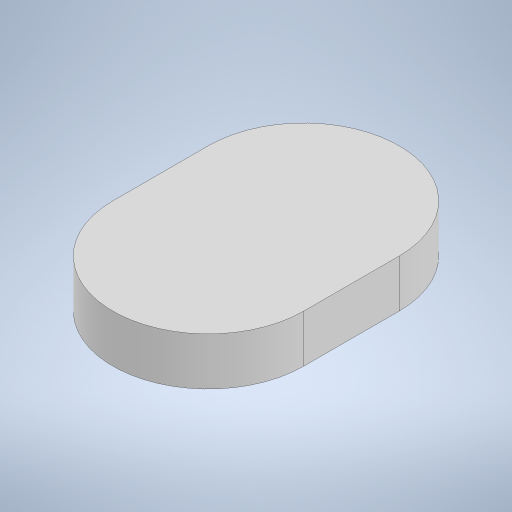
# Autodesk Inventor part: glosnik
Saved by Autodesk Inventor 2024.3 (Build 283343000, 343)
## iProperties
Created: 2025-03-17
Part Number: glosnik
Material: Generic
Document SubType Name: Modeling
Designer: eleme
Density: 1 g/cm^3
Appearance: Default
Author: eleme
Autodesk Inventor part; units mm, degrees
ref_plane "YZ Plane" through (0, 0, 0) normal (1, 0, 0) x (0, 1, 0)
ref_plane "XZ Plane" through (0, 0, 0) normal (0, 1, 0) x (-1, 0, 0)
ref_plane "XY Plane" through (0, 0, 0) normal (0, 0, 1) x (1, 0, 0)
sketch "Sketch1" plane through (0, 0, 0) normal (0, 1, 0) x (-1, 0, 0)
  line L0 (0, 0) -> (20, 0)
  line L1 (20, 0) -> (20, 30)
  line L2 (20, 30) -> (0, 30)
  line L3 (0, 30) -> (0, 0)
  line L4 (0, 30) -> (20, 0)
  line L5 (0, 0) -> (20, 30)
  line L6 (11.5, 3.5) -> (8.5, 3.5)
  line L7 (3.5, 8.5) -> (3.5, 21.5)
  line L8 (8.5, 26.5) -> (11.5, 26.5)
  line L9 (16.5, 21.5) -> (16.5, 8.5)
  line L10 (16.5, 3.5) -> (3.5, 26.5) construction
  line L11 (3.5, 3.5) -> (16.5, 26.5) construction
  arc A0 (8.5, 26.5) -> (3.5, 21.5) centre (8.5, 21.5) ccw
  arc A1 (16.5, 21.5) -> (11.5, 26.5) centre (11.5, 21.5) ccw
  arc A2 (11.5, 3.5) -> (16.5, 8.5) centre (11.5, 8.5) ccw
  arc A3 (3.5, 8.5) -> (8.5, 3.5) centre (8.5, 8.5) ccw
  line L12 (12.5954, 0) -> (7.0954, 0)
  line L13 (7.0954, 0) -> (7.0954, 1.5)
  line L14 (7.0954, 1.5) -> (12.5954, 1.5)
  line L15 (12.5954, 1.5) -> (12.5954, 0)
  point P0 (10, 15)
  dimension "d0" = 20
  dimension "d1" = 30
  dimension "d5" = 13
  dimension "d6" = 23
  dimension "d7" = 5
  dimension "d10" = 5.5
  dimension "d11" = 1.5
  constraints: 32 end point, 9 point on line, 8 point on circle, 8 tangent, 6 parallel, 4 centre point, 3 equal radius, 3 horizontal, 3 midpoint, 3 perpendicular
  measures "d0" distance of L2.end L1.end
  measures "d1" distance of L1.end L0.end
  measures "d5" distance of L10.end L11.end
  measures "d6" distance of L11.start L10.end
  measures "d7" radius of A0
  measures "d10" distance of L13.end L14.end
  measures "d11" distance of L12.end L13.end
extrude "Extrusion1" add sketch "Sketch1" along normal blind 5
fillet "Fillet1" radius 10 4 edges at (0, 2.5, 30) (0, 2.5, 0) (-20, 2.5, 0) (-20, 2.5, 30)
extrude "Extrusion2" cut sketch "Sketch1" along normal blind 1 contours A3 L7 A0 L4 L5 | L5 L4 A2 L6 A3 | A0 L8 A1 L5 L4 | L5 A1 L9 A2 L4
body "Solid1"
